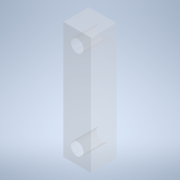
# Autodesk Inventor part: plateplummer
Saved by Autodesk Inventor 2021 (Build 250183000, 183)
## iProperties
Created: 2023-10-29
Part Number: plateplummer
Material: PMMA Plastic
Document SubType Name: Modeling
Designer: M
Density: 1.24028 g/cm^3
Appearance: Polycarbonate - Clear
Mass: 9.8 g
Surface Area: 34.0129 cm^2
Volume: 7.90142 cm^3
Author: M
Autodesk Inventor part; units mm, degrees
ref_plane "YZ Plane" through (0, 0, 0) normal (1, 0, 0) x (0, 1, 0)
ref_plane "XZ Plane" through (0, 0, 0) normal (0, 1, 0) x (-1, 0, 0)
ref_plane "XY Plane" through (0, 0, 0) normal (0, 0, 1) x (1, 0, 0)
sketch "Sketch1" plane through (0, 0, 0) normal (0, 0, 1) x (1, 0, 0)
  line L0 (0, 55) -> (13, 55)
  line L1 (13, 55) -> (13, 0)
  line L2 (13, 0) -> (0, 0)
  line L3 (0, 0) -> (0, 55)
  circle A0 centre (6.5, 48.5) radius 3
  circle A1 centre (6.5, 6.5) radius 3
  line L4 (6.5, 48.5) -> (6.5, 6.5)
  dimension "d2" = 6
  dimension "d3" = 6
  dimension "d4" = 42
  dimension "d5" = 55
  dimension "d6" = 13
  dimension "d7" = 6.5
  dimension "d8" = 6.5
  constraints: 10 end point, 2 centre point, 2 parallel, 1 coincident, 1 horizontal, 1 perpendicular, 1 vertical
  measures "d2" diameter of A1
  measures "d3" diameter of A0
  measures "d4" distance of L4.start L4.end
  measures "d5" distance of L2.end L0.start
  measures "d6" distance of L0.start L0.end
  measures "d7" distance between parallel lines of L3 L4
  measures "d8" distance from line of L0 L4.start
extrude "Extrusion1" add sketch "Sketch1" along normal blind 12
equation "\"d3\" = d2"
equation "\"d7\" = 0.5 * d6"
equation "\"d8\" = -0.5 * d4 + 0.5 * d5"
body "Solid1"
